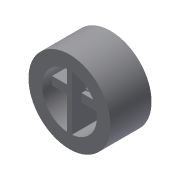
# Autodesk Inventor part: Mount
Saved by Autodesk Inventor 2014 SP1 (Build 180222100, 222)
## iProperties
Created: 2015-04-12
Part Number: Mount
Material: Generic
Document SubType Name: Modeling
Designer: Citrus CAD
Mass: 1.06718 g
Surface Area: 10.579 cm^2
Volume: 1.06718 cm^3
Density: 1 g/cm^3
Appearance: Default
Author: Citrus CAD
Autodesk Inventor part; units mm, degrees
ref_plane "YZ Plane" through (0, 0, 0) normal (1, 0, 0) x (0, 1, 0)
ref_plane "XZ Plane" through (0, 0, 0) normal (0, 1, 0) x (-1, 0, 0)
ref_plane "XY Plane" through (0, 0, 0) normal (0, 0, 1) x (1, 0, 0)
sketch "Sketch1" plane through (0, 0, 0) normal (1, 0, 0) x (0, 1, 0)
  line L0 (-7.62, 2.54) -> (0, 2.54)
  line L1 (0, 2.54) -> (0, 0)
  line L2 (0, 0) -> (-7.62, 0)
  line L3 (-7.62, 0) -> (-7.62, 2.54)
  line L4 (-7.62, 7.62) -> (-5.08, 7.62)
  line L5 (-5.08, 7.62) -> (-5.08, 2.54)
  line L6 (-5.08, 2.54) -> (-7.62, 2.54)
  line L7 (-7.62, 2.54) -> (-7.62, 7.62)
  line L8 (-1.27, 5.08) -> (0, 5.08)
  line L9 (0, 5.08) -> (0, 2.54)
  line L10 (0, 2.54) -> (-1.27, 2.54)
  line L11 (-1.27, 2.54) -> (-1.27, 5.08)
  dimension "d0" = 7.62
  dimension "d1" = 2.54
  dimension "d2" = 5.08
  dimension "d3" = 2.54
  dimension "d4" = 1.27
  dimension "d5" = 2.54
  constraints: 24 end point, 6 parallel, 3 horizontal, 3 perpendicular, 1 coincident
  measures "d0" distance of L1.end L2.end
  measures "d1" distance of L2.end L0.start
  measures "d2" distance of L0.start L4.start
  measures "d3" distance of L4.start L4.end
  measures "d4" distance of L8.start L8.end
  measures "d5" distance of L8.end L0.end
revolve "Revolution1" add sketch "Sketch1" angle 360 about axis through (0, 0, 2.54) along (0, 0, -1)
sketch "Sketch2" plane through (0, 0, 2.54) normal (0, 0, 1) x (1, 0, 0)
  circle A0 centre (-2.9748, -2.859) radius 0.3175
  line L0 (-0.6666, -1.081) -> (-1.7631, -2.859) construction
  line L1 (-1.7631, -2.859) -> (-2.9748, -2.859) construction
  circle A1 centre (0, 0) radius 1.27 construction
  circle A2 centre (-1.7631, -2.859) radius 0.3175
  point P0 (0, 0)
  dimension "d7" = 0.635
  dimension "d8" = 1.778
  dimension "d9" = 0.635
  constraints: 4 end point, 2 centre point, 2 coincident, 1 point on line, 2 other
  measures "d7" diameter of A0
  measures "d8" vertical distance of L0.start L0.end
  measures "d9" diameter of A2
extrude "Extrusion1" cut sketch "Sketch2" along normal mid plane 25.4
sketch "Sketch3" plane through (0, 0, 2.54) normal (0, 0, 1) x (1, 0, 0)
  line L0 (0, 0) -> (1.8228, -2.926) construction
  line L1 (1.8228, -2.926) -> (3.0389, -2.926) construction
  line L2 (-1.5657, -3.1077) -> (1.8228, -2.926) construction
  circle A0 centre (-1.7631, -2.859) radius 0.3175 projected
  circle A1 centre (1.8228, -2.926) radius 0.3175
  circle A2 centre (3.0389, -2.926) radius 0.3175
  circle A3 centre (1.962, 2.9682) radius 0.3175
  circle A4 centre (3.1781, 2.9682) radius 0.3175
  circle A5 centre (-1.2085, 2.832) radius 0.3175
  circle A6 centre (-2.506, 2.8679) radius 0.3175
  point P0 (0, 0)
  dimension "d12" = 0.635
  dimension "d13" = 0.635
  dimension "d14" = 0.635
  dimension "d15" = 0.635
  dimension "d16" = 0.635
  dimension "d17" = 0.635
  constraints: 6 centre point, 6 end point, 1 coincident, 2 other
  measures "d12" diameter of A1
  measures "d13" diameter of A2
  measures "d14" diameter of A3
  measures "d15" diameter of A4
  measures "d16" diameter of A5
  measures "d17" diameter of A6
extrude "Extrusion2" cut sketch "Sketch3" along normal mid plane 25.4 contours A1 | A2 | A3 | A4 | A5 | A6
sketch "Sketch4" plane through (0, 0, 2.54) normal (0, 0, 1) x (1, 0, 0)
  line L0 (-0.4549, -6.2616) -> (0.4549, -6.2616)
  line L1 (0.4549, -6.2616) -> (0.4549, 6.2616)
  line L2 (0.4549, 6.2616) -> (-0.4549, 6.2616)
  line L3 (-0.4549, 6.2616) -> (-0.4549, -6.2616)
  line L4 (-0.4549, -6.2616) -> (0.4549, 6.2616) construction
  line L5 (0.4549, -6.2616) -> (-0.4549, 6.2616) construction
  point P0 (0, 0)
  point P1 (0, 0)
  constraints: 12 end point, 2 midpoint, 2 parallel, 1 horizontal, 1 perpendicular
extrude "Extrusion3" add sketch "Sketch4" along normal blind 5.08
sketch "Sketch5" plane through (0, 0, 2.54) normal (0, 0, 1) x (1, 0, 0)
  line L0 (-6.9573, 0.776) -> (6.9573, 0.776)
  line L1 (6.9573, 0.776) -> (6.9573, -0.776)
  line L2 (6.9573, -0.776) -> (-6.9573, -0.776)
  line L3 (-6.9573, -0.776) -> (-6.9573, 0.776)
  line L4 (-6.9573, 0.776) -> (6.9573, -0.776) construction
  line L5 (6.9573, 0.776) -> (-6.9573, -0.776) construction
  point P0 (0, 0)
  point P1 (0, 0)
  constraints: 12 end point, 2 midpoint, 2 parallel, 1 horizontal, 1 perpendicular
extrude "Extrusion4" add sketch "Sketch5" along normal blind 3.302
body "Solid1"
